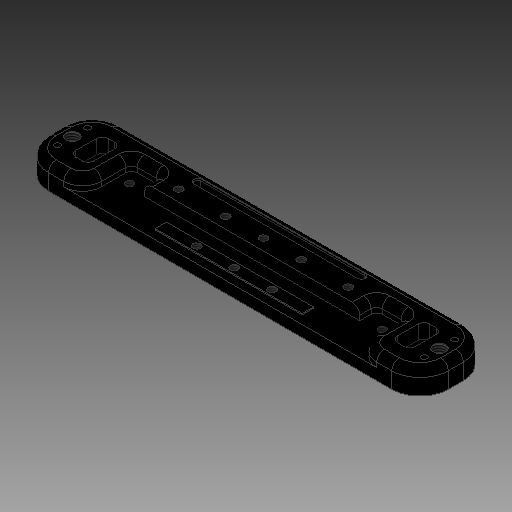
# Autodesk Inventor part: LR Hard Plate
Saved by Autodesk Inventor 2019 (Build 230136000, 136)
## iProperties
Created: 2016-01-25
Part Number: LR Hard Plate
Material: Aluminum 6061
Document SubType Name: Modeling
Designer: IEUser
Density: 2.7 g/cm^3
Appearance: Anodized - Black
Mass: 189.289 g
Surface Area: 256.318 cm^2
Volume: 70.1071 cm^3
Author: IEUser
Autodesk Inventor part; units mm, degrees
ref_plane "YZ Plane" through (0, 0, 0) normal (1, 0, 0) x (0, 1, 0)
ref_plane "XZ Plane" through (0, 0, 0) normal (0, 1, 0) x (-1, 0, 0)
ref_plane "XY Plane" through (0, 0, 0) normal (0, 0, 1) x (1, 0, 0)
sketch "Body Outline" plane through (0, 0, 0) normal (0, 1, 0) x (-1, 0, 0)
  line L0 (106, -19) -> (-106, -19)
  line L1 (-106, -19) -> (-106, 19)
  line L2 (-106, 19) -> (106, 19)
  line L3 (106, 19) -> (106, -19)
  point P0 (0, 0)
  dimension "d0" = 212
  dimension "d1" = 106
  dimension "d2" = 38
  dimension "d3" = 19
  constraints: 8 end point, 2 parallel, 1 horizontal, 1 perpendicular
  measures "d0" distance of L0.start L0.end
  measures "d1" distance from line of point (0, 0) L3
  measures "d2" distance of L0.end L1.end
  measures "d3" distance from line of L0 point (0, 0)
extrude "Body" add sketch "Body Outline" along normal blind 12.5
sketch "Metal Band Cutout Outline" plane through (0, 12.5, 0) normal (0, 1, 0) x (1, 0, 0)
  line L0 (-73, -19) -> (-73, 7)
  line L1 (-73, 7) -> (-57, 7)
  line L2 (-57, 7) -> (-57, -2)
  line L3 (-57, -2) -> (57, -2)
  line L4 (57, -2) -> (57, 7)
  line L5 (57, 7) -> (73, 7)
  line L6 (73, 7) -> (73, -19)
  line L7 (73, -19) -> (-73, -19)
  line L8 (-106, -19) -> (106, -19) projected
  point P0 (0, 0)
  dimension "d6" = 146
  dimension "d7" = 73
  dimension "d8" = 0
  dimension "d9" = 114
  dimension "d10" = 17
  dimension "d11" = 26
  dimension "d12" = 26
  dimension "d13" = 16
  constraints: 16 end point, 7 perpendicular, 1 vertical
  measures "d6" distance between parallel lines of L6 L0
  measures "d7" distance from line of point (0, 0) L0
  measures "d8" distance between parallel lines of L8 L7
  measures "d9" distance between parallel lines of L4 L2
  measures "d10" distance between parallel lines of L7 L3
  measures "d11" distance between parallel lines of L7 L1
  measures "d12" distance between parallel lines of L8 L5
  measures "d13" distance of L0.end L1.end
extrude "Metal Band Cutout" cut sketch "Metal Band Cutout Outline" against normal blind 6.5
sketch "Metal Band Clamp Outline" plane through (0, 6, 0) normal (0, 1, 0) x (1, 0, 0)
  line L0 (-39, -8.5) -> (39, -8.5)
  line L1 (39, -8.5) -> (39, -14.5)
  line L2 (39, -14.5) -> (-39, -14.5)
  line L3 (-39, -14.5) -> (-39, -8.5)
  line L4 (73, -19) -> (-73, -19) projected
  point P0 (0, 0)
  dimension "d16" = 39
  dimension "d17" = 78
  dimension "d18" = 6
  dimension "d19" = 4.5
  constraints: 8 end point, 2 parallel, 1 horizontal, 1 perpendicular
  measures "d16" distance from line of point (0, 0) L3
  measures "d17" distance of L1.end L2.end
  measures "d18" distance of L2.end L0.start
  measures "d19" distance between parallel lines of L4 L2
extrude "Metal Band Clamp" add sketch "Metal Band Clamp Outline" along normal blind 0.6
sketch "Lower Skin Passage Outline" plane through (0, 12.5, 0) normal (0, 1, 0) x (1, 0, 0)
  line L0 (-45, 14.1) -> (45, 14.1)
  line L1 (45, 14.1) -> (45, 10.9)
  line L2 (45, 10.9) -> (-45, 10.9)
  line L3 (-45, 10.9) -> (-45, 14.1)
  line L4 (106, 19) -> (-106, 19) projected
  point P0 (0, 0)
  dimension "d22" = 3.2
  dimension "d23" = 4.9
  dimension "d24" = 90
  dimension "d25" = 45
  constraints: 8 end point, 2 parallel, 1 horizontal, 1 perpendicular
  measures "d22" distance of L2.end L0.start
  measures "d23" distance between parallel lines of L4 L0
  measures "d24" distance of L0.start L0.end
  measures "d25" distance from line of point (0, 0) L3
extrude "Lower Skin Passage" cut sketch "Lower Skin Passage Outline" against normal through all
sketch "Rail Cutouts Outline" plane through (0, 12.5, 0) normal (0, 1, 0) x (1, 0, 0)
  line L0 (-90.05, 8.55) -> (-80.45, 8.55)
  line L1 (-80.45, 8.55) -> (-80.45, -8.55)
  line L2 (-80.45, -8.55) -> (-90.05, -8.55)
  line L3 (-90.05, -8.55) -> (-90.05, 8.55)
  line L4 (-106, 19) -> (-106, -19) projected
  line L5 (80.45, 8.55) -> (90.05, 8.55)
  line L6 (90.05, 8.55) -> (90.05, -8.55)
  line L7 (90.05, -8.55) -> (80.45, -8.55)
  line L8 (80.45, -8.55) -> (80.45, 8.55)
  line L9 (106, -19) -> (106, 19) projected
  point P0 (0, 0)
  dimension "d28" = 17.1
  dimension "d29" = 9.6
  dimension "d30" = 15.95
  dimension "d31" = 8.55
  dimension "d32" = 9.6
  dimension "d33" = 17.1
  dimension "d34" = 8.55
  dimension "d35" = 15.95
  constraints: 16 end point, 4 parallel, 2 horizontal, 2 perpendicular
  measures "d28" distance of L2.end L0.start
  measures "d29" distance of L0.start L0.end
  measures "d30" distance between parallel lines of L4 L3
  measures "d31" distance from line of point (0, 0) L0
  measures "d32" distance of L5.start L5.end
  measures "d33" distance of L5.end L6.end
  measures "d34" distance from line of point (0, 0) L5
  measures "d35" distance between parallel lines of L9 L6
extrude "Rail Cutouts" cut sketch "Rail Cutouts Outline" against normal blind 7.5
sketch "Dowel Pin Hole Positions" plane through (0, 12.5, 0) normal (0, 1, 0) x (1, 0, 0)
  line L0 (-106, 19) -> (-106, -19) projected
  line L1 (106, 19) -> (106, -19) projected
  point P0 (0, 0)
  point P1 (-97.35, 8)
  point P2 (-97.35, -8)
  point P3 (97.35, 8)
  point P4 (97.35, -8)
  dimension "d38" = 8.65
  dimension "d39" = 8.65
  dimension "d40" = 8.65
  dimension "d41" = 8.65
  dimension "d42" = 8
  dimension "d43" = 8
  dimension "d44" = 8
  dimension "d45" = 8
  measures "d38" distance from line of L0 point (-97.35, 8)
  measures "d39" distance from line of L0 point (-97.35, -8)
  measures "d40" distance from line of L1 point (97.35, 8)
  measures "d41" distance from line of L1 point (97.35, -8)
  measures "d42" vertical distance of point (0, 0) point (-97.35, 8)
  measures "d43" vertical distance of point (0, 0) point (-97.35, -8)
  measures "d44" vertical distance of point (97.35, -8) point (0, 0)
  measures "d45" vertical distance of point (0, 0) point (97.35, 8)
hole "Dowel Pin Holes" at (-97.35, 12.5, -8) at (-97.35, 12.5, 8) at (97.35, 12.5, -8) at (97.35, 12.5, 8) direction (0, -1, 0) diameter 2 end through all counterbore diameter 3.1 counterbore depth 8
sketch "Fastening Hole Positions" plane through (0, 0, 0) normal (0, -1, 0) x (1, 0, 0)
  line L0 (-106, 19) -> (-106, -19) projected
  line L1 (106, -19) -> (106, 19) projected
  point P0 (0, 0)
  point P1 (-97.35, 0)
  point P2 (97.35, 0)
  dimension "d95" = 8.65
  dimension "d96" = 8.65
  dimension "d97" = 0
  dimension "d98" = 0
  measures "d95" distance from line of L0 point (-97.35, 0)
  measures "d96" distance from line of L1 point (97.35, 0)
  measures "d97" vertical distance of point (0, 0) point (97.35, 0)
  measures "d98" vertical distance of point (0, 0) point (-97.35, 0)
hole "Fastening Holes" at (-97.35, 0, 0) at (97.35, 0, 0) direction (0, 1, 0) diameter 6.647 end through all thread size "M8x1.25" class "6H" standard "ISO Metric profile"
sketch "Clamp Hole Positions" plane through (0, 0, 0) normal (0, -1, 0) x (1, 0, 0)
  line L0 (106, 19) -> (-106, 19) projected
  line L1 (-106, -19) -> (106, -19) projected
  point P0 (0, 0)
  point P1 (45, -4)
  point P2 (20, -4)
  point P3 (0, -4)
  point P4 (-20, -4)
  point P5 (-45, -4)
  point P6 (67, 0)
  point P7 (-67, 0)
  point P8 (-20, 11.5)
  point P9 (20, 11.5)
  point P10 (0, 11.5)
  dimension "d53" = 7.5
  dimension "d54" = 7.5
  dimension "d55" = 7.5
  dimension "d56" = 0
  dimension "d57" = 20
  dimension "d58" = 20
  dimension "d59" = 15
  dimension "d60" = 15
  dimension "d61" = 15
  dimension "d62" = 15
  dimension "d63" = 15
  dimension "d64" = 0
  dimension "d65" = 20
  dimension "d66" = 20
  dimension "d67" = 25
  dimension "d68" = 25
  dimension "d69" = 67
  dimension "d70" = 67
  dimension "d71" = 0
  dimension "d72" = 0
  measures "d53" distance from line of L0 point (20, 11.5)
  measures "d54" distance from line of L0 point (0, 11.5)
  measures "d55" distance from line of L0 point (-20, 11.5)
  measures "d56" horizontal distance of point (0, 0) point (0, 11.5)
  measures "d57" distance of point (0, 11.5) point (20, 11.5)
  measures "d58" distance of point (-20, 11.5) point (0, 11.5)
  measures "d59" distance from line of L1 point (45, -4)
  measures "d60" distance from line of L1 point (20, -4)
  measures "d61" distance from line of L1 point (0, -4)
  measures "d62" distance from line of L1 point (-20, -4)
  measures "d63" distance from line of L1 point (-45, -4)
  measures "d64" horizontal distance of point (0, 0) point (0, -4)
  measures "d65" distance of point (-20, -4) point (0, -4)
  measures "d66" distance of point (20, -4) point (0, -4)
  measures "d67" distance of point (45, -4) point (20, -4)
  measures "d68" distance of point (-45, -4) point (-20, -4)
  measures "d69" distance of point (0, 0) point (67, 0)
  measures "d70" distance of point (0, 0) point (-67, 0)
  measures "d71" vertical distance of point (0, 0) point (67, 0)
  measures "d72" vertical distance of point (0, 0) point (-67, 0)
hole "Clamp Holes" at (45, 0, -4) at (20, 0, -4) at (0, 0, -4) at (-20, 0, -4) at (-45, 0, -4) at (67, 0, 0) at (-67, 0, 0) at (-20, 0, 11.5) at (20, 0, 11.5) at (0, 0, 11.5) direction (0, 1, 0) diameter 4.134 end through all thread size "M5x0.8" class "6H" standard "ISO Metric profile"
sketch "Rail Hole Positions" plane through (0, 0, 0) normal (0, -1, 0) x (1, 0, 0)
  point P0 (0, 0)
  point P1 (85.25, 4.5)
  point P2 (85.25, -4.5)
  point P3 (-85.25, -4.5)
  point P4 (-85.25, 4.5)
  dimension "d80" = 85.25
  dimension "d81" = 85.25
  dimension "d82" = 85.25
  dimension "d83" = 85.25
  dimension "d84" = 4.5
  dimension "d85" = 4.5
  dimension "d86" = 4.5
  dimension "d87" = 4.5
  measures "d80" horizontal distance of point (0, 0) point (85.25, -4.5)
  measures "d81" horizontal distance of point (0, 0) point (85.25, 4.5)
  measures "d82" horizontal distance of point (0, 0) point (-85.25, 4.5)
  measures "d83" horizontal distance of point (0, 0) point (-85.25, -4.5)
  measures "d84" vertical distance of point (0, 0) point (85.25, -4.5)
  measures "d85" vertical distance of point (0, 0) point (85.25, 4.5)
  measures "d86" vertical distance of point (0, 0) point (-85.25, 4.5)
  measures "d87" vertical distance of point (-85.25, -4.5) point (0, 0)
hole "Rail Holes" at (85.25, 0, 4.5) at (85.25, 0, -4.5) at (-85.25, 0, -4.5) at (-85.25, 0, 4.5) direction (0, 1, 0) diameter 5.1 end through all
fillet "Body Fillet" radius 15 4 edges at (-106, 6.25, 19) (-106, 6.25, -19) (106, 6.25, -19) (106, 6.25, 19)
fillet "Body Fillet" radius 10 2 edges at (-73, 9.25, 19) (73, 9.25, 19)
fillet "Body Fillet" radius 3 12 edges at (-80.45, 8.75, -8.55) (-90.05, 8.75, -8.55) (-90.05, 8.75, 8.55) (-80.45, 8.75, 8.55) (-57, 9.25, -7) (-73, 9.25, -7) (73, 9.25, -7) (57, 9.25, -7) (90.05, 8.75, -8.55) (80.45, 8.75, -8.55) (80.45, 8.75, 8.55) (90.05, 8.75, 8.55)
fillet "Body Fillet" radius 4 11 edges at (-57, 12.5, -2.5) (-65, 12.5, -7) (-73, 12.5, 6) (-89.5, 12.5, 19) (-106, 12.5, 0) (0, 12.5, -19) (106, 12.5, 0) (89.5, 12.5, 19) (73, 12.5, 6) (65, 12.5, -7) (57, 12.5, -2.5)
fillet "Body Fillet" radius 1.6 4 edges at (45, 6.25, -14.1) (-45, 6.25, -14.1) (-45, 6.25, -10.9) (45, 6.25, -10.9)
chamfer "Lower Skin Passage Chamfer" distance 0.5 angle 45 4 edges at (0, 12.5, -14.1) (0, 12.5, -10.9) (0, 0, -14.1) (0, 0, -10.9)
equation "\"d1\" = 0.5 * d0"
equation "\"d3\" = 0.5 * d2"
equation "\"d7\" = 0.5 * d6"
equation "\"d16\" = 0.5 * d17"
equation "\"d25\" = 0.5 * d24"
equation "\"d31\" = 0.5 * d28"
equation "\"d32\" = d29"
equation "\"d33\" = d28"
equation "\"d34\" = d31"
equation "\"d35\" = d30"
equation "\"d39\" = d38"
equation "\"d40\" = d38"
equation "\"d41\" = d38"
equation "\"d43\" = d42"
equation "\"d44\" = d42"
equation "\"d45\" = d42"
equation "\"d96\" = d95"
equation "\"d54\" = d53"
equation "\"d55\" = d53"
equation "\"d60\" = d59"
equation "\"d61\" = d59"
equation "\"d62\" = d59"
equation "\"d63\" = d59"
equation "\"d65\" = d66"
equation "\"d68\" = d67"
equation "\"d70\" = d69"
equation "\"d81\" = d80"
equation "\"d82\" = d80"
equation "\"d83\" = d80"
equation "\"d85\" = d84"
equation "\"d86\" = d84"
equation "\"d87\" = d84"
body "Solid1"
